# Autodesk Inventor part: DIN41612
Saved by Autodesk Inventor 2015 SP1 (Build 190203100, 203)
## iProperties
Created: 2015-06-25
Part Number: DIN41612
Material: Generic
Document SubType Name: Modeling
Designer: Patrick
Density: 1 g/cm^3
Appearance: DIN41612_32, DIN41612
Author: Patrick
Autodesk Inventor part; units mm, degrees
ref_plane "YZ Plane" through (0, 0, 0) normal (1, 0, 0) x (0, 1, 0)
ref_plane "XZ Plane" through (0, 0, 0) normal (0, 1, 0) x (-1, 0, 0)
ref_plane "XY Plane" through (0, 0, 0) normal (0, 0, 1) x (1, 0, 0)
sketch "DIN41612_32, DIN41612_6" plane through (0, 0, 0) normal (0, 0, 1) x (1, 0, 0)
  line L0 (-6.25, -27.1) -> (-6.25, 27.1)
  line L1 (-6.25, 27.1) -> (7.95, 27.1)
  line L2 (7.95, 27.1) -> (7.95, -27.1)
  line L3 (7.95, -27.1) -> (-6.25, -27.1)
  constraints: 8 end point
extrude "Extrusion1" add sketch "DIN41612_32, DIN41612_6" along normal blind 1
body "Solid1"
